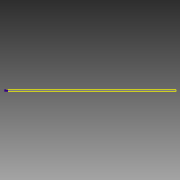
# Autodesk Inventor part: ledstrip-60led-5050
Saved by Autodesk Inventor 2013 (Build 170138000, 138)
## iProperties
Created: 2013-03-07
Part Number: ledstrip-60led-5050
Material: Generic
Document SubType Name: Modeling
Designer: Beth Scott
Density: 1 g/cm^3
Author: Beth Scott
Autodesk Inventor part; units mm, degrees
ref_plane "YZ Plane" through (0, 0, 0) normal (1, 0, 0) x (0, 1, 0)
ref_plane "XZ Plane" through (0, 0, 0) normal (0, 1, 0) x (-1, 0, 0)
ref_plane "XY Plane" through (0, 0, 0) normal (0, 0, 1) x (1, 0, 0)
sketch "PCB_Pad" plane through (0, 0, 0) normal (0, 0, 1) x (1, 0, 0)
  circle A0 centre (6.811, 24.8402) radius 0.375
  arc A1 (6.186, 25.7152) -> (6.186, 23.9652) centre (6.186, 24.8402) ccw
  line L0 (6.186, 25.7152) -> (7.436, 25.7152)
  line L1 (6.186, 23.9652) -> (7.436, 23.9652)
  arc A2 (7.436, 23.9652) -> (7.436, 25.7152) centre (7.436, 24.8402) ccw
  line L2 (6.811, 25.7152) -> (6.811, 23.9652) construction
  line L3 (5.311, 24.8402) -> (8.311, 24.8402) construction
  point P0 (6.811, 24.8402)
  dimension "d12" = 3
  dimension "d13" = 0.75
  dimension "d14" = 1.75
  measures "d12" distance of L3.start L3.end
  measures "d13" diameter of A0
  measures "d14" distance of L2.start L2.end
sketch "PCB_Pad_Group" plane through (0, 0, 0) normal (0, 0, 1) x (1, 0, 0)
  circle A0 centre (6.4629, 25.645) radius 0.375
  arc A1 (5.8379, 26.52) -> (5.8379, 24.77) centre (5.8379, 25.645) ccw
  line L0 (5.8379, 26.52) -> (7.0879, 26.52)
  line L1 (5.8379, 24.77) -> (7.0879, 24.77)
  arc A2 (7.0879, 24.77) -> (7.0879, 26.52) centre (7.0879, 25.645) ccw
  line L2 (6.4629, 26.52) -> (6.4629, 24.77) construction
  line L3 (4.9629, 25.645) -> (7.9629, 25.645) construction
  circle A3 centre (10.0629, 25.645) radius 0.375
  arc A4 (9.4379, 26.52) -> (9.4379, 24.77) centre (9.4379, 25.645) ccw
  line L4 (9.4379, 26.52) -> (10.6879, 26.52)
  line L5 (9.4379, 24.77) -> (10.6879, 24.77)
  arc A5 (10.6879, 24.77) -> (10.6879, 26.52) centre (10.6879, 25.645) ccw
  line L6 (10.0629, 26.52) -> (10.0629, 24.77) construction
  line L7 (8.5629, 25.645) -> (11.5629, 25.645) construction
  circle A6 centre (10.0629, 22.645) radius 0.375
  arc A7 (9.4379, 23.52) -> (9.4379, 21.77) centre (9.4379, 22.645) ccw
  line L8 (9.4379, 23.52) -> (10.6879, 23.52)
  line L9 (9.4379, 21.77) -> (10.6879, 21.77)
  arc A8 (10.6879, 21.77) -> (10.6879, 23.52) centre (10.6879, 22.645) ccw
  line L10 (10.0629, 23.52) -> (10.0629, 21.77) construction
  line L11 (8.5629, 22.645) -> (11.5629, 22.645) construction
  circle A9 centre (10.0629, 19.645) radius 0.375
  arc A10 (9.4379, 20.52) -> (9.4379, 18.77) centre (9.4379, 19.645) ccw
  line L12 (9.4379, 20.52) -> (10.6879, 20.52)
  line L13 (9.4379, 18.77) -> (10.6879, 18.77)
  arc A11 (10.6879, 18.77) -> (10.6879, 20.52) centre (10.6879, 19.645) ccw
  line L14 (10.0629, 20.52) -> (10.0629, 18.77) construction
  line L15 (8.5629, 19.645) -> (11.5629, 19.645) construction
  circle A12 centre (6.4629, 19.645) radius 0.375
  arc A13 (5.8379, 20.52) -> (5.8379, 18.77) centre (5.8379, 19.645) ccw
  line L16 (5.8379, 20.52) -> (7.0879, 20.52)
  line L17 (5.8379, 18.77) -> (7.0879, 18.77)
  arc A14 (7.0879, 18.77) -> (7.0879, 20.52) centre (7.0879, 19.645) ccw
  line L18 (6.4629, 20.52) -> (6.4629, 18.77) construction
  line L19 (4.9629, 19.645) -> (7.9629, 19.645) construction
  circle A15 centre (6.4629, 22.645) radius 0.375
  arc A16 (5.8379, 23.52) -> (5.8379, 21.77) centre (5.8379, 22.645) ccw
  line L20 (5.8379, 23.52) -> (7.0879, 23.52)
  line L21 (5.8379, 21.77) -> (7.0879, 21.77)
  arc A17 (7.0879, 21.77) -> (7.0879, 23.52) centre (7.0879, 22.645) ccw
  line L22 (6.4629, 23.52) -> (6.4629, 21.77) construction
  line L23 (4.9629, 22.645) -> (7.9629, 22.645) construction
  point P0 (8.2629, 22.645)
  dimension "d15" = 3
  dimension "d16" = 3
  dimension "d17" = 3.6
sketch "1m_Outline" plane through (0, 0, 0) normal (0, 0, 1) x (1, 0, 0)
  line L0 (0, 0) -> (1000, 0)
  line L1 (1000, 0) -> (1000, 10)
  line L2 (1000, 10) -> (0, 10)
  line L3 (0, 10) -> (0, 0)
  line L4 (0, 5) -> (1000, 5) construction
  point P0 (500.9843, 5)
  dimension "d0" = 1000
  dimension "d1" = 10
  measures "d0" distance of L2.end L1.end
  measures "d1" distance of L1.end L0.end
sketch "LED_5050" plane through (0, 0, 0) normal (0, 0, 1) x (1, 0, 0)
  line L0 (7.6271, 7.5) -> (12.6271, 7.5)
  line L1 (12.6271, 7.5) -> (12.6271, 2.5)
  line L2 (12.6271, 2.5) -> (7.6271, 2.5)
  line L3 (7.6271, 2.5) -> (7.6271, 7.5)
  line L4 (7.6271, 7.5) -> (12.6271, 7.5)
  line L5 (12.6271, 7.5) -> (12.6271, 9)
  line L6 (12.6271, 9) -> (7.6271, 9)
  line L7 (7.6271, 9) -> (7.6271, 7.5)
  line L8 (7.6271, 2.5) -> (12.6271, 2.5)
  line L9 (12.6271, 2.5) -> (12.6271, 1)
  line L10 (12.6271, 1) -> (7.6271, 1)
  line L11 (7.6271, 1) -> (7.6271, 2.5)
  point P0 (10.0557, 4.9286)
  point P1 (7.6271, 5)
  dimension "d2" = 5
  dimension "d3" = 5
  dimension "d5" = 1.5
  measures "d2" distance of L1.end L8.start
  measures "d3" distance of L4.end L1.end
  measures "d5" distance of L4.end L5.end
sketch "Cap_1206" plane through (0, 0, 0) normal (0, 0, 1) x (1, 0, 0)
  line L0 (14.0271, 6.6) -> (15.6271, 6.6)
  line L1 (15.6271, 6.6) -> (15.6271, 3.4)
  line L2 (15.6271, 3.4) -> (14.0271, 3.4)
  line L3 (14.0271, 3.4) -> (14.0271, 6.6)
  line L4 (14.0271, 6.6) -> (15.6271, 6.6)
  line L5 (15.6271, 6.6) -> (15.6271, 8.1)
  line L6 (15.6271, 8.1) -> (14.0271, 8.1)
  line L7 (14.0271, 8.1) -> (14.0271, 6.6)
  line L8 (14.0271, 3.4) -> (15.6271, 3.4)
  line L9 (15.6271, 3.4) -> (15.6271, 1.9)
  line L10 (15.6271, 1.9) -> (14.0271, 1.9)
  line L11 (14.0271, 1.9) -> (14.0271, 3.4)
  point P0 (14.8692, 5)
  point P1 (14.0271, 5)
  dimension "d6" = 1.6
  dimension "d7" = 3.2
  measures "d6" distance of L1.end L2.end
  measures "d7" distance of L0.end L1.end
sketch "LED_Repeating_Unit" plane through (0, 0, 0) normal (0, 0, 1) x (1, 0, 0)
  circle A0 centre (18.0271, 8) radius 0.375
  arc A1 (17.4021, 8.875) -> (17.4021, 7.125) centre (17.4021, 8) ccw
  line L0 (17.4021, 8.875) -> (18.6521, 8.875)
  line L1 (17.4021, 7.125) -> (18.6521, 7.125)
  arc A2 (18.6521, 7.125) -> (18.6521, 8.875) centre (18.6521, 8) ccw
  line L2 (18.0271, 8.875) -> (18.0271, 7.125) construction
  line L3 (16.5271, 8) -> (19.5271, 8) construction
  circle A3 centre (21.6271, 8) radius 0.375
  arc A4 (21.0021, 8.875) -> (21.0021, 7.125) centre (21.0021, 8) ccw
  line L4 (21.0021, 8.875) -> (22.2521, 8.875)
  line L5 (21.0021, 7.125) -> (22.2521, 7.125)
  arc A5 (22.2521, 7.125) -> (22.2521, 8.875) centre (22.2521, 8) ccw
  line L6 (21.6271, 8.875) -> (21.6271, 7.125) construction
  line L7 (20.1271, 8) -> (23.1271, 8) construction
  circle A6 centre (21.6271, 5) radius 0.375
  arc A7 (21.0021, 5.875) -> (21.0021, 4.125) centre (21.0021, 5) ccw
  line L8 (21.0021, 5.875) -> (22.2521, 5.875)
  line L9 (21.0021, 4.125) -> (22.2521, 4.125)
  arc A8 (22.2521, 4.125) -> (22.2521, 5.875) centre (22.2521, 5) ccw
  line L10 (21.6271, 5.875) -> (21.6271, 4.125) construction
  line L11 (20.1271, 5) -> (23.1271, 5) construction
  circle A9 centre (21.6271, 2) radius 0.375
  arc A10 (21.0021, 2.875) -> (21.0021, 1.125) centre (21.0021, 2) ccw
  line L12 (21.0021, 2.875) -> (22.2521, 2.875)
  line L13 (21.0021, 1.125) -> (22.2521, 1.125)
  arc A11 (22.2521, 1.125) -> (22.2521, 2.875) centre (22.2521, 2) ccw
  line L14 (21.6271, 2.875) -> (21.6271, 1.125) construction
  line L15 (20.1271, 2) -> (23.1271, 2) construction
  circle A12 centre (18.0271, 2) radius 0.375
  arc A13 (17.4021, 2.875) -> (17.4021, 1.125) centre (17.4021, 2) ccw
  line L16 (17.4021, 2.875) -> (18.6521, 2.875)
  line L17 (17.4021, 1.125) -> (18.6521, 1.125)
  arc A14 (18.6521, 1.125) -> (18.6521, 2.875) centre (18.6521, 2) ccw
  line L18 (18.0271, 2.875) -> (18.0271, 1.125) construction
  line L19 (16.5271, 2) -> (19.5271, 2) construction
  circle A15 centre (18.0271, 5) radius 0.375
  arc A16 (17.4021, 5.875) -> (17.4021, 4.125) centre (17.4021, 5) ccw
  line L20 (17.4021, 5.875) -> (18.6521, 5.875)
  line L21 (17.4021, 4.125) -> (18.6521, 4.125)
  arc A17 (18.6521, 4.125) -> (18.6521, 5.875) centre (18.6521, 5) ccw
  line L22 (18.0271, 5.875) -> (18.0271, 4.125) construction
  line L23 (16.5271, 5) -> (19.5271, 5) construction
  line L24 (7.6271, 7.5) -> (12.6271, 7.5)
  line L25 (12.6271, 7.5) -> (12.6271, 2.5)
  line L26 (12.6271, 2.5) -> (7.6271, 2.5)
  line L27 (7.6271, 2.5) -> (7.6271, 7.5)
  line L28 (7.6271, 7.5) -> (12.6271, 7.5)
  line L29 (12.6271, 7.5) -> (12.6271, 9)
  line L30 (12.6271, 9) -> (7.6271, 9)
  line L31 (7.6271, 9) -> (7.6271, 7.5)
  line L32 (7.6271, 2.5) -> (12.6271, 2.5)
  line L33 (12.6271, 2.5) -> (12.6271, 1)
  line L34 (12.6271, 1) -> (7.6271, 1)
  line L35 (7.6271, 1) -> (7.6271, 2.5)
  line L36 (14.0271, 6.6) -> (15.6271, 6.6)
  line L37 (15.6271, 6.6) -> (15.6271, 3.4)
  line L38 (15.6271, 3.4) -> (14.0271, 3.4)
  line L39 (14.0271, 3.4) -> (14.0271, 6.6)
  line L40 (14.0271, 6.6) -> (15.6271, 6.6)
  line L41 (15.6271, 6.6) -> (15.6271, 8.1)
  line L42 (15.6271, 8.1) -> (14.0271, 8.1)
  line L43 (14.0271, 8.1) -> (14.0271, 6.6)
  line L44 (14.0271, 3.4) -> (15.6271, 3.4)
  line L45 (15.6271, 3.4) -> (15.6271, 1.9)
  line L46 (15.6271, 1.9) -> (14.0271, 1.9)
  line L47 (14.0271, 1.9) -> (14.0271, 3.4)
  point P0 (14.9174, 4.9762)
  dimension "d18" = 8
  dimension "d19" = 15.5
sketch "Flex-PCB" plane through (0, 0, 0) normal (0, 1, 0) x (-1, 0, 0)
  line L0 (0, -5) -> (1000, -5)
  line L1 (1000, -5) -> (1000, 5)
  line L2 (1000, 5) -> (0, 5)
  line L3 (0, 5) -> (0, -5)
  line L4 (0, 0) -> (1000, 0) construction
  constraints: 1 other
extrude "Flex-PCB Extrusion" add sketch "Flex-PCB" along normal blind 0.3
sketch "Sketch3" plane through (0, 0.3, 0) normal (0, 1, 0) x (1, 0, 0)
  line L0 (0, 5) -> (-1000, 5) projected
  line L1 (-1000, 5) -> (-1000, -5) projected
  line L2 (-1000, -5) -> (0, -5) projected
  line L3 (0, -5) -> (0, 5) projected
  line L4 (0, 0) -> (6.1653, 0) construction
  circle A0 centre (-2.1, 3) radius 0.375
  arc A1 (-2.725, 3.875) -> (-2.725, 2.125) centre (-2.725, 3) ccw
  line L5 (-2.725, 3.875) -> (-1.475, 3.875)
  line L6 (-2.725, 2.125) -> (-1.475, 2.125)
  arc A2 (-1.475, 2.125) -> (-1.475, 3.875) centre (-1.475, 3) ccw
  line L7 (-2.1, 3.875) -> (-2.1, 2.125) construction
  line L8 (-3.6, 3) -> (-0.6, 3) construction
  circle A3 centre (1.5, 3) radius 0.375
  arc A4 (0.875, 3.875) -> (0.875, 2.125) centre (0.875, 3) ccw
  line L9 (0.875, 3.875) -> (2.125, 3.875)
  line L10 (0.875, 2.125) -> (2.125, 2.125)
  arc A5 (2.125, 2.125) -> (2.125, 3.875) centre (2.125, 3) ccw
  line L11 (1.5, 3.875) -> (1.5, 2.125) construction
  line L12 (0, 3) -> (3, 3) construction
  circle A6 centre (1.5, 0) radius 0.375
  arc A7 (0.875, 0.875) -> (0.875, -0.875) centre (0.875, 0) ccw
  line L13 (0.875, 0.875) -> (2.125, 0.875)
  line L14 (0.875, -0.875) -> (2.125, -0.875)
  arc A8 (2.125, -0.875) -> (2.125, 0.875) centre (2.125, 0) ccw
  line L15 (1.5, 0.875) -> (1.5, -0.875) construction
  line L16 (0, 0) -> (3, 0) construction
  circle A9 centre (1.5, -3) radius 0.375
  arc A10 (0.875, -2.125) -> (0.875, -3.875) centre (0.875, -3) ccw
  line L17 (0.875, -2.125) -> (2.125, -2.125)
  line L18 (0.875, -3.875) -> (2.125, -3.875)
  arc A11 (2.125, -3.875) -> (2.125, -2.125) centre (2.125, -3) ccw
  line L19 (1.5, -2.125) -> (1.5, -3.875) construction
  line L20 (0, -3) -> (3, -3) construction
  circle A12 centre (-2.1, -3) radius 0.375
  arc A13 (-2.725, -2.125) -> (-2.725, -3.875) centre (-2.725, -3) ccw
  line L21 (-2.725, -2.125) -> (-1.475, -2.125)
  line L22 (-2.725, -3.875) -> (-1.475, -3.875)
  arc A14 (-1.475, -3.875) -> (-1.475, -2.125) centre (-1.475, -3) ccw
  line L23 (-2.1, -2.125) -> (-2.1, -3.875) construction
  line L24 (-3.6, -3) -> (-0.6, -3) construction
  circle A15 centre (-2.1, 0) radius 0.375
  arc A16 (-2.725, 0.875) -> (-2.725, -0.875) centre (-2.725, 0) ccw
  line L25 (-2.725, 0.875) -> (-1.475, 0.875)
  line L26 (-2.725, -0.875) -> (-1.475, -0.875)
  arc A17 (-1.475, -0.875) -> (-1.475, 0.875) centre (-1.475, 0) ccw
  line L27 (-2.1, 0.875) -> (-2.1, -0.875) construction
  line L28 (-3.6, 0) -> (-0.6, 0) construction
  line L29 (-12.5, 2.5) -> (-7.5, 2.5)
  line L30 (-7.5, 2.5) -> (-7.5, -2.5)
  line L31 (-7.5, -2.5) -> (-12.5, -2.5)
  line L32 (-12.5, -2.5) -> (-12.5, 2.5)
  line L33 (-12.5, 2.5) -> (-7.5, 2.5)
  line L34 (-7.5, 2.5) -> (-7.5, 4)
  line L35 (-7.5, 4) -> (-12.5, 4)
  line L36 (-12.5, 4) -> (-12.5, 2.5)
  line L37 (-12.5, -2.5) -> (-7.5, -2.5)
  line L38 (-7.5, -2.5) -> (-7.5, -4)
  line L39 (-7.5, -4) -> (-12.5, -4)
  line L40 (-12.5, -4) -> (-12.5, -2.5)
  line L41 (-6.1, 1.6) -> (-4.5, 1.6)
  line L42 (-4.5, 1.6) -> (-4.5, -1.6)
  line L43 (-4.5, -1.6) -> (-6.1, -1.6)
  line L44 (-6.1, -1.6) -> (-6.1, 1.6)
  line L45 (-6.1, 1.6) -> (-4.5, 1.6)
  line L46 (-4.5, 1.6) -> (-4.5, 3.1)
  line L47 (-4.5, 3.1) -> (-6.1, 3.1)
  line L48 (-6.1, 3.1) -> (-6.1, 1.6)
  line L49 (-6.1, -1.6) -> (-4.5, -1.6)
  line L50 (-4.5, -1.6) -> (-4.5, -3.1)
  line L51 (-4.5, -3.1) -> (-6.1, -3.1)
  line L52 (-6.1, -3.1) -> (-6.1, -1.6)
  constraints: 2 end point, 2 horizontal, 1 midpoint, 1 other
body "Solid2"
